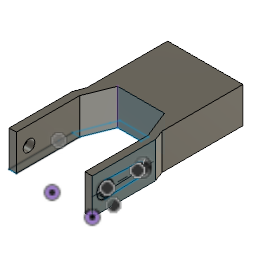
Wrist (Autodesk Fusion 360 design; units mm, degrees)
part number: 2026-08-08-17-19-53-385
Autodesk Fusion 360 part; units mm, degrees
sketch "Sketch1" plane through (0, 0, 0) normal (0, 0, 1) x (1, 0, 0)
  line L0 (-16.25, -0.6886) -> (-16.25, 29.3114)
  line L1 (-16.25, 29.3114) -> (-19.75, 29.3114)
  line L2 (-19.75, 29.3114) -> (-19.75, -0.6886)
  line L3 (-19.75, -0.6886) -> (-16.25, -0.6886)
  spline S0 degree 3 poles (-19.7481, 22.9091) (-19.7487, 22.9276) (-19.7494, 22.9461) (-19.75, 22.9645) knots 0 0 0 0 0.001755 0.001755 0.001755 0.001755
  line L4 (-16.25, 29.3114) -> (-11.1067, 42.1478)
  line L5 (-11.1067, 42.1478) -> (0, 42.1478)
  line L6 (0, 42.1478) -> (0, 45.6478)
  line L7 (-14.7933, 42.3572) -> (-13.4749, 45.6478)
  line L8 (-13.4749, 45.6478) -> (0, 45.6478)
  line L9 (-19.75, 29.3114) -> (-14.7933, 42.3572)
  dimension "d1" = 3.5
  dimension "d2" = 16.25
  dimension "d3" = 30
  dimension "d8" = -3.5
  constraint vertical L0
  constraint perpendicular L0 L1
  constraint perpendicular L1 L2
  constraint perpendicular L0 L3
  constraint coincident L2 S0.end
  constraint perpendicular L0 L5
  constraint perpendicular L5 L6
  measures "d1" distance of L0.start L2.end
  measures "d2" distance of origin L0
  measures "d3" distance of L0.start L0.end
extrude "Extrude1" add sketch "Sketch1" along normal blind 12 contours L0 L1 L2 L3 S0
extrude "Extrude2" add sketch "Sketch1" along normal blind 17
mirror "Mirror1" about plane through (0, 0, 0) normal (1, 0, 0) of bodies 1 merged
sketch "Sketch2" plane through (19.75, 0, 0) normal (1, 0, 0) x (0, 1, 0)
  line L0 (-0.6886, 0) -> (29.3114, 0)
  line L1 (29.3114, 0) -> (29.3114, 17)
  line L2 (29.3114, 17) -> (-0.6886, 17)
  line L3 (-0.6886, 17) -> (-0.6886, 0)
  line L4 (-0.6886, 8.5) -> (29.3114, 8.5) construction
  line L5 (23.3114, 9.6158) -> (23.3114, 7.3842) construction
  line L6 (5.3214, 12.3) -> (5.8374, 12.2634)
  circle A0 centre (5.3114, 8.5) radius 3.8
  arc A1 (20.7878, 5.3) -> (20.9673, 11.695) centre (20.7889, 8.5) ccw
  line L7 (20.9673, 11.695) -> (5.3214, 12.3)
  line L8 (20.7878, 5.3) -> (5.3209, 4.7)
  point P0 (9.3621, 0)
  point P1 (23.3114, 8.5)
  point P2 (6.3843, 8.5)
  dimension "d31" = 6
  dimension "d32" = 18
  dimension "d40" = 7.6
  dimension "d45" = 3.2
  constraint coincident L0 P0
  constraint midpoint L3 L4.start
  constraint midpoint L1 L4.end
  constraint midpoint L5 P1
  constraint coincident L4 P1
  constraint perpendicular L4 L5
  constraint coincident L4 P2
  constraint coincident A0 L6.start
  constraint coincident L4 A1.centre
  constraint coincident L6.end A0
  constraint coincident L8.end A0
  constraint coincident L4 A0.centre
  measures "d31" distance of L3 A0.centre
  measures "d32" distance of L5 A0.centre
  measures "d40" diameter of A0
  measures "d45" radius of A1
sketch "Sketch4" plane through (0, 42.1478, 0) normal (0, -1, 0) x (1, 0, 0)
  line L0 (-11.1067, 0) -> (11.1067, 0)
  line L1 (11.1067, 0) -> (11.1067, 17)
  line L2 (11.1067, 17) -> (-11.1067, 17)
  line L3 (-11.1067, 17) -> (-11.1067, 0)
sketch "Sketch5" plane through (0, 45.6478, 0) normal (0, 1, 0) x (-1, 0, 0)
  line L0 (-13.4749, 0) -> (13.4749, 0)
  line L1 (13.4749, 0) -> (13.4749, 17)
  line L2 (13.4749, 17) -> (-13.4749, 17)
  line L3 (-13.4749, 17) -> (-13.4749, 0)
extrude "Extrude7" cut sketch "Sketch2" against normal blind 1.5 from surface at -2 contours L6 A0 L7 | L6 A0 L8
extrude "Extrude8" cut sketch "Sketch2" against normal blind 4 contours L6 A0 L7 | L6 A0 L8 | A0 L7 | A0 L8
extrude "Extrude9" cut sketch "Sketch2" against normal blind 2.5 contours A0 A1 L7 L8
sketch "Sketch6" plane through (-19.75, 0, 0) normal (-1, 0, 0) x (0, -1, 0)
  line L0 (-29.3114, 0) -> (0.6886, 0)
  line L1 (0.6886, 0) -> (0.6886, 17)
  line L2 (0.6886, 17) -> (-29.3114, 17)
  line L3 (-29.3114, 17) -> (-29.3114, 0)
  circle A0 centre (-5.3114, 8.5) radius 2.75
  line L4 (-29.3114, 0) -> (0.6886, 0)
  point P0 (0.6886, 8.5)
  dimension "d49" = 5.5
  dimension "d52" = 6
  dimension "d53" = 8.5
  measures "d49" diameter of A0
  measures "d52" horizontal distance of A0.centre P0
  measures "d53" distance of A0.centre L4
extrude "Extrude10" cut sketch "Sketch6" against normal blind 4 contours A0
extrude "Extrude11" add sketch "Sketch5" along normal blind 5
move_face "OffsetFaces1" offset 4.4 2 faces at (13.4749, 47.3145, 11.3333) (-13.4749, 48.9811, 11.3333)
sketch "Sketch14" plane through (0, 50.6478, 0) normal (0, 1, 0) x (-1, 0, 0)
  line L0 (-17.8749, 17) -> (-17.8749, 0)
  line L1 (-17.8749, 0) -> (17.8749, 0)
  line L2 (17.8749, 0) -> (17.8749, 17)
  line L3 (17.8749, 17) -> (-17.8749, 17)
  line L4 (0, 17) -> (0, 0) construction
  line L5 (11.8356, 2.35) -> (-11.8356, 2.35) construction
  line L6 (-11.8356, 2.35) -> (-11.8356, 14.65) construction
  line L7 (-11.8356, 14.65) -> (11.8356, 14.65) construction
  line L8 (11.8356, 14.65) -> (11.8356, 2.35) construction
  line L9 (11.875, 2.325) -> (11.875, 14.675) construction
  line L10 (13.4749, 0) -> (0, 0) construction
  line L11 (11.875, 14.675) -> (-11.875, 14.675) construction
  line L12 (-11.875, 14.675) -> (11.875, 14.675)
  line L13 (11.875, 14.675) -> (11.875, 2.325)
  line L14 (11.875, 2.325) -> (-11.875, 2.325)
  line L15 (-11.875, 2.325) -> (-11.875, 14.675)
  line L16 (-17.8749, 17) -> (-17.8749, 0)
  line L17 (-17.8749, 0) -> (17.8749, 0)
  line L18 (17.8749, 0) -> (17.8749, 17)
  line L19 (17.8749, 17) -> (-17.8749, 17)
  dimension "d99" = 5.9999
  dimension "d100" = 2.35
  dimension "d101" = 23.75
  constraint midpoint L3 L4.start
  constraint coincident L4.end L10.end
  constraint horizontal L5
  constraint perpendicular L5 L6
  constraint parallel L5 L7
  constraint parallel L6 L8
  constraint horizontal L12
  constraint vertical L13
  constraint horizontal L14
  constraint vertical L15
  constraint coincident L9.start L13.end
  constraint coincident L11.end L12.start
  measures "d99" distance of L2 L9
  measures "d100" distance of L5 L10
  measures "d101" distance of L9.end L11.end
extrude "Extrude17" add sketch "Sketch14" along normal blind 22
sketch "Sketch15" plane through (0, 72.6478, 0) normal (0, 1, 0) x (-1, 0, 0)
  line L0 (11.875, 2.325) -> (-11.875, 2.325)
  line L1 (-11.875, 2.325) -> (-11.875, 14.675)
  line L2 (-11.875, 14.675) -> (11.875, 14.675)
  line L3 (11.875, 14.675) -> (11.875, 2.325)
  line L4 (17.8749, 17) -> (-17.8749, 17)
  line L5 (-17.8749, 17) -> (-17.8749, 0)
  line L6 (-17.8749, 0) -> (17.8749, 0)
  line L7 (17.8749, 0) -> (17.8749, 17)
  circle A0 centre (14.325, 8.5) radius 1
  line L8 (0, 2.325) -> (0, 14.675) construction
  circle A1 centre (-14.325, 8.5) radius 1
  dimension "d104" = 2
  dimension "d106" = 2.45
  constraint midpoint L0 L8.start
  constraint midpoint L2 L8.end
  constraint symmetric A0 L8 A1
  measures "d104" diameter of A0
  measures "d106" distance of L3 A0.centre
extrude "Extrude18" cut sketch "Sketch15" against normal blind 10 contours A0 | A1
